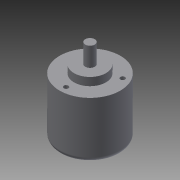
# Autodesk Inventor part: rotary encoder
Saved by Autodesk Inventor 2014 (Build 180170000, 170)
## iProperties
Created: 2015-12-28
Part Number: rotary encoder
Material: Generic
Document SubType Name: Modeling
Designer: RMcComber
Density: 1 g/cm^3
Appearance: Default
Author: RMcComber
Autodesk Inventor part; units mm, degrees
ref_plane "YZ Plane" through (0, 0, 0) normal (1, 0, 0) x (0, 1, 0)
ref_plane "XZ Plane" through (0, 0, 0) normal (0, 1, 0) x (-1, 0, 0)
ref_plane "XY Plane" through (0, 0, 0) normal (0, 0, 1) x (1, 0, 0)
sketch "Sketch1" plane through (0, 0, 0) normal (0, 0, 1) x (1, 0, 0)
  circle A0 centre (0, 0) radius 15 construction
  line L0 (0, 0) -> (-12.9904, 7.5) construction
  line L1 (0, 0) -> (12.9904, 7.5) construction
  line L2 (0, 0) -> (0, -15) construction
  circle A1 centre (-12.9904, 7.5) radius 1.45
  circle A2 centre (12.9904, 7.5) radius 1.45
  circle A3 centre (0, -15) radius 1.45
  circle A4 centre (0, 0) radius 3 construction
  circle A5 centre (0, 0) radius 19
  dimension "d0" = 120
  dimension "d1" = 120
  dimension "d2" = 120
  dimension "d3" = 2.9
  dimension "d4" = 6
  dimension "d5" = 15
  dimension "d6" = 30
  dimension "d7" = 38
  constraints: 6 centre point, 6 coincident, 6 end point, 3 point on circle, 2 equal radius, 1 vertical
  measures "d0" angle of L0 L2
  measures "d1" angle of L1 L2
  measures "d2" angle of L1 L0
  measures "d3" diameter of A1
  measures "d4" diameter of A4
  measures "d5" distance of L0.end A4.centre
  measures "d6" diameter of A0
  measures "d7" diameter of A5
extrude "Extrusion1" add sketch "Sketch1" against normal blind 10
sketch "Sketch2" plane through (0, 0, -10) normal (0, 0, -1) x (-1, 0, 0)
  circle A0 centre (0, 0) radius 19 projected
extrude "Extrusion2" add sketch "Sketch2" along normal blind 25.25
fillet "Fillet1" radius 3 1 edges at (19, 0, -35.25)
sketch "Sketch3" plane through (0, 0, 0) normal (0, 0, 1) x (1, 0, 0)
  circle A0 centre (0, 0) radius 19 projected
  circle A1 centre (0, 0) radius 10
  dimension "d13" = 20
  constraints: 1 centre point, 1 coincident
  measures "d13" diameter of A1
extrude "Extrusion3" add sketch "Sketch3" along normal blind 5 contours A1
sketch "Sketch4" plane through (0, 0, 5) normal (0, 0, 1) x (1, 0, 0)
  circle A0 centre (0, 0) radius 10 projected
  circle A1 centre (0, 0) radius 3
  dimension "d16" = 6
  constraints: 1 centre point, 1 coincident
  measures "d16" diameter of A1
extrude "Extrusion4" add sketch "Sketch4" along normal blind 12 contours A1
equation "\"d1\" = d0"
body "Solid1"
